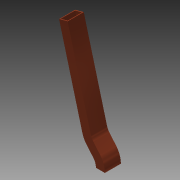
# Autodesk Inventor part: bendy bit
Saved by Autodesk Inventor 2015 (Build 190159000, 159)
## iProperties
Created: 2014-05-21
Part Number: bendy bit
Material: Copper
Document SubType Name: Modeling
Designer: jad211
Density: 8.94 g/cm^3
Appearance: Copper - Satin
Author: jad211
Autodesk Inventor part; units mm, degrees
ref_plane "YZ Plane" through (0, 0, 0) normal (1, 0, 0) x (0, 1, 0)
ref_plane "XZ Plane" through (0, 0, 0) normal (0, 1, 0) x (-1, 0, 0)
ref_plane "XY Plane" through (0, 0, 0) normal (0, 0, 1) x (1, 0, 0)
sketch "Sketch1" plane through (0, 0, 0) normal (0, 1, 0) x (-1, 0, 0)
  line L0 (0, 0) -> (9.899, 0)
  line L1 (9.899, 0) -> (9.899, -17.799)
  line L2 (9.899, -17.799) -> (0, -17.799)
  line L3 (0, -17.799) -> (0, 0)
  line L4 (1, -1) -> (8.899, -1)
  line L5 (8.899, -1) -> (8.899, -16.799)
  line L6 (8.899, -16.799) -> (1, -16.799)
  line L7 (1, -16.799) -> (1, -1)
  dimension "d8" = 1
  dimension "d9" = 1
  dimension "d10" = 1
  dimension "d11" = 1
  dimension "d12" = 7.899
  dimension "d13" = 15.799
  constraints: 16 end point
  measures "d8" distance between parallel lines of L0 L4
  measures "d9" distance between parallel lines of L2 L6
  measures "d10" distance between parallel lines of L3 L7
  measures "d11" distance between parallel lines of L1 L5
  measures "d12" distance of L5.end L6.end
  measures "d13" distance of L6.end L4.start
sketch "Sketch2" plane through (0, 0, 0) normal (0, 0, 1) x (1, 0, 0)
  arc A0 (0, 0) -> (-5.4679, 14.8499) centre (-22.899, 0) ccw
  line L0 (-5.4679, 14.8499) -> (-12.6935, 23.3315)
  line L1 (0, 0) -> (-22.899, 0) construction
  line L2 (-19.2837, 4.8137) -> (-24.9164, 25.8353) construction
  line L3 (-7.0614, 29.3682) -> (4.2878, -12.9875) construction
  arc A1 (-15.3547, 28.3973) -> (-12.6935, 23.3315) centre (-2.7977, 31.762) ccw
  line L4 (-24.9164, 25.8353) -> (-15.3547, 28.3973) construction
  line L5 (-24.928, 64.1254) -> (-15.3547, 28.3973) construction
  line L6 (-15.3547, 28.3973) -> (-41.2366, 124.9899)
  line L7 (0, 0) -> (-38.1419, -10.2201) construction
  line L8 (-2.7977, 31.762) -> (5.3302, 1.4282) construction
  line L9 (-22.899, 0) -> (-32.2813, 35.0152) construction
  line L10 (-41.2366, 124.9899) -> (-73.5917, 116.3204) construction
  dimension "d7" = 18.161
  dimension "d14" = 9.899
  dimension "d15" = 15
  dimension "d16" = 31.404
  dimension "d17" = 13
  dimension "d18" = 22.899
  dimension "d21" = 100
  constraints: 22 end point, 5 parallel, 4 point on circle, 4 tangent, 2 centre point, 2 perpendicular, 2 point on line, 1 horizontal
  measures "d7" distance between parallel lines of L3 L2
  measures "d14" distance of L2.end L4.end
  measures "d15" angle of L1 L4
  measures "d17" distance from line of L4.end L8
  measures "d18" distance between parallel lines of L3 L9
  measures "d21" distance between parallel lines of L4 L10
sweep "Sweep1" add profiles "Sketch1" path "Sketch2"
equation "\"d8\" = d11"
equation "\"d9\" = d11"
equation "\"d10\" = d11"
body "Solid1"
